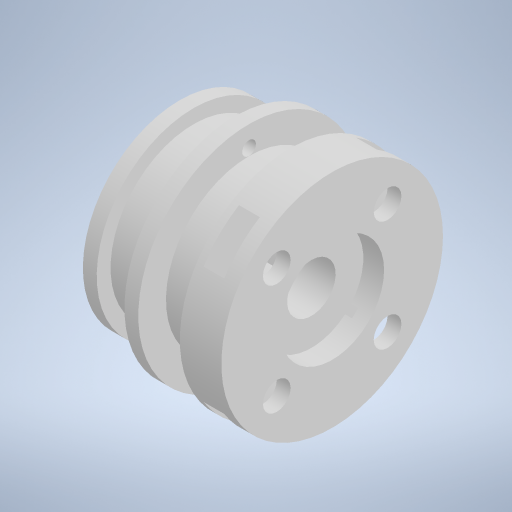
# Autodesk Inventor part: Spool 24mm
Saved by Autodesk Inventor 2023 (Build 270158000, 158)
## iProperties
Created: 2022-10-10
Part Number: Spool 24mm
Material: Generic
Document SubType Name: Modeling
Designer: deli
Density: 1 g/cm^3
Appearance: Default
Author: deli
Autodesk Inventor part; units mm, degrees
ref_plane "YZ Plane" through (0, 0, 0) normal (1, 0, 0) x (0, 1, 0)
ref_plane "XZ Plane" through (0, 0, 0) normal (0, 1, 0) x (-1, 0, 0)
ref_plane "XY Plane" through (0, 0, 0) normal (0, 0, 1) x (1, 0, 0)
sketch "Sketch1" plane through (0, 0, 0) normal (1, 0, 0) x (0, 1, 0)
  circle A0 centre (13.6363, 26.4679) radius 14
  circle A1 centre (13.6363, 26.4679) radius 3.5
  point P0 (0, 0)
  dimension "d0" = 28
  dimension "d1" = 7
  constraints: 2 centre point, 1 coincident
  measures "d0" diameter of A0
  measures "d1" diameter of A1
extrude "Extrusion1" add sketch "Sketch1" along normal blind 2
sketch "Sketch2" plane through (2, 13.6363, 26.4679) normal (1, 0, 0) x (0, 0, -1)
  circle A0 centre (0, 0) radius 3.5 projected
  circle A1 centre (0, 0) radius 12
  point P0 (26.4679, -13.6363)
  dimension "d4" = 24
  constraints: 1 centre point, 1 coincident
  measures "d4" diameter of A1
extrude "Extrusion2" add sketch "Sketch2" along normal blind 6
sketch "Sketch3" plane through (8, 13.6363, 26.4679) normal (1, 0, 0) x (0, 0, -1)
  circle A0 centre (0, 0) radius 3.5 projected
  circle A1 centre (0, 0) radius 12 construction
  circle A2 centre (0, 13) radius 1
  circle A3 centre (0, 0) radius 16
  point P0 (26.4679, -13.6363)
  dimension "d11" = 2
  dimension "d12" = 0
  dimension "d31" = 32
  constraints: 2 centre point, 1 coincident, 1 tangent
  measures "d11" diameter of A2
  measures "d12" horizontal distance of A2.centre A0.centre
  measures "d31" diameter of A3
extrude "Extrusion3" add sketch "Sketch3" along normal blind 2
sketch "Sketch4" plane through (10, 13.6363, 26.4679) normal (1, 0, 0) x (0, 0, -1)
  circle A0 centre (0, 0) radius 12 projected
  circle A1 centre (0, 0) radius 3.5 projected
  point P0 (26.4679, -13.6363)
extrude "Extrusion4" add sketch "Sketch4" along normal blind 6
sketch "Sketch5" plane through (16, 13.6363, 26.4679) normal (1, 0, 0) x (0, 0, -1)
  circle A0 centre (0, 0) radius 3.5 projected
  circle A1 centre (0, 0) radius 16
  point P0 (26.4679, -13.6363)
  dimension "d30" = 32
  constraints: 1 centre point, 1 coincident
  measures "d30" diameter of A1
extrude "Extrusion5" add sketch "Sketch5" along normal blind 6
ref_plane "Work Plane1" through (17, 13.6363, 26.4679) normal (-1, 0, 0) x (0, 0, 1)
sketch "Sketch7" plane through (17, 13.6363, 26.4679) normal (-1, 0, 0) x (0, 0, 1)
  circle A0 centre (0, 0) radius 3.5 projected
  circle A1 centre (0, 0) radius 16
  circle A2 centre (-8, 8) radius 4.125 construction
  circle A3 centre (8, 8) radius 4.125 construction
  circle A4 centre (8, -8) radius 4.125 construction
  circle A5 centre (-8, -8) radius 4.125 construction
  circle A6 centre (0, 0) radius 7.1887 construction
  line L0 (-8, 8) -> (8, 8) construction
  line L1 (8, 8) -> (8, -8) construction
  line L2 (8, -8) -> (-8, -8) construction
  line L3 (-8, -8) -> (-8, 8) construction
  line L4 (-8.4563, 13.5828) -> (-3.9568, 9.0834)
  line L5 (-3.9568, 9.0834) -> (-5.0402, 5.0402)
  line L6 (-5.0402, 5.0402) -> (-9.0834, 3.9568)
  line L7 (-9.0834, 3.9568) -> (-13.5828, 8.4563)
  line L8 (-12.0432, 6.9166) -> (-10.9598, 10.9598)
  line L9 (-10.9598, 10.9598) -> (-6.9166, 12.0432)
  line L10 (6.9166, 12.0432) -> (10.9598, 10.9598)
  line L11 (10.9598, 10.9598) -> (12.0432, 6.9166)
  line L12 (13.5828, 8.4563) -> (9.0834, 3.9568)
  line L13 (9.0834, 3.9568) -> (5.0402, 5.0402)
  line L14 (5.0402, 5.0402) -> (3.9568, 9.0834)
  line L15 (3.9568, 9.0834) -> (8.4563, 13.5828)
  line L16 (9.0834, -3.9568) -> (13.5828, -8.4563)
  line L17 (12.0432, -6.9166) -> (10.9598, -10.9598)
  line L18 (10.9598, -10.9598) -> (6.9166, -12.0432)
  line L19 (8.4563, -13.5828) -> (3.9568, -9.0834)
  line L20 (3.9568, -9.0834) -> (5.0402, -5.0402)
  line L21 (5.0402, -5.0402) -> (9.0834, -3.9568)
  line L22 (-3.9568, -9.0834) -> (-8.4563, -13.5828)
  line L23 (-6.9166, -12.0432) -> (-10.9598, -10.9598)
  line L24 (-10.9598, -10.9598) -> (-12.0432, -6.9166)
  line L25 (-13.5828, -8.4563) -> (-9.0834, -3.9568)
  line L26 (-9.0834, -3.9568) -> (-5.0402, -5.0402)
  line L27 (-5.0402, -5.0402) -> (-3.9568, -9.0834)
  point P0 (-26.4679, -13.6363)
  dimension "d32" = 32
  dimension "d16" = 8.25
  dimension "d17" = 16
  dimension "d18" = 7.25
  constraints: 56 end point, 9 point on line, 5 centre point, 5 coincident, 4 tangent, 3 equal length, 3 equal radius, 2 collinear, 1 parallel, 1 perpendicular, 1 vertical, 62 other
  measures "d16" diameter of A2
  measures "d17" distance of L0.start L0.end
  measures "d18" distance between parallel lines of L4 L7
extrude "Extrusion6" cut sketch "Sketch7" against normal blind 3 contours L12 L11 L10 L15 A1 | A1 L19 L18 L17 L16 | L12 L13 L14 L15 L10 L11 | L17 L18 L19 L20 L21 L16 | L4 L9 L8 L7 A1 | A1 L25 L24 L23 L22 | L4 L5 L6 L7 L8 L9 | L23 L24 L25 L26 L27 L22
sketch "Sketch8" plane through (22, 13.6363, 26.4679) normal (1, 0, 0) x (0, 0, -1)
  circle A0 centre (0, 0) radius 9.3137 construction
  circle A1 centre (-8, 8) radius 2
  circle A2 centre (8, 8) radius 2
  circle A3 centre (8, -8) radius 2
  circle A4 centre (-8, -8) radius 2
  line L0 (-8, 8) -> (8, 8) construction
  line L1 (8, 8) -> (8, -8) construction
  line L2 (8, -8) -> (-8, -8) construction
  line L3 (-8, -8) -> (-8, 8) construction
  circle A5 centre (0, 0) radius 3.5 construction
  circle A6 centre (0, 0) radius 7.5
  point P0 (26.4679, -13.6363)
  dimension "d21" = 4
  dimension "d22" = 16
  dimension "d23" = 15
  constraints: 8 end point, 6 centre point, 4 tangent, 3 equal radius, 3 perpendicular, 1 coincident, 1 concentric, 1 vertical
  measures "d21" diameter of A4
  measures "d22" distance of L0.start L0.end
  measures "d23" diameter of A6
extrude "Extrusion7" cut sketch "Sketch8" against normal blind 3 contours A6
sketch "Sketch9" plane through (22, 13.6363, 26.4679) normal (1, 0, 0) x (0, 0, -1)
  circle A0 centre (-8, 8) radius 2
  circle A1 centre (8, 8) radius 2
  circle A2 centre (8, -8) radius 2
  circle A3 centre (-8, -8) radius 2
  line L0 (-8, 8) -> (8, 8) construction
  line L1 (8, 8) -> (8, -8) construction
  line L2 (8, -8) -> (-8, -8) construction
  line L3 (-8, -8) -> (-8, 8) construction
  circle A4 centre (0, 0) radius 9.3137 construction
  circle A5 centre (0, 0) radius 3.5 construction
  point P0 (26.4679, -13.6363)
  dimension "d26" = 4
  dimension "d27" = 16
  constraints: 8 end point, 5 centre point, 4 perpendicular, 3 equal radius, 3 tangent, 1 concentric, 1 horizontal
  measures "d26" diameter of A0
  measures "d27" distance of L0.start L0.end
extrude "Extrusion8" cut sketch "Sketch9" against normal blind 3
body "Solid1"
